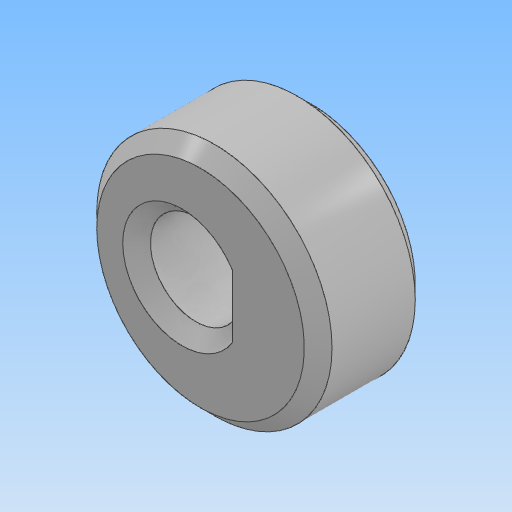
# Autodesk Inventor part: V1_Cycloid_Cam
Saved by Autodesk Inventor 2021 (Build 250183000, 183)
## iProperties
Created: 2020-12-17
Part Number: V1_Cycloid_Cam
Material: PPS Plastic
Document SubType Name: Modeling
Designer: ndevr
Density: 1.637 g/cm^3
Appearance: Smooth - White
Author: ndevr
Autodesk Inventor part; units mm, degrees
ref_plane "Work Plane19" through (-1.0583, 0, 0) normal (1, 0, 0) x (0, 0, 1)
ref_plane "XZ Vertical Span" through (0, 0, 0) normal (0, 1, 0) x (-1, 0, 0)
derived "V1_N17Cycloid_CamShaft.ipt"
sketch "Sketch16" plane through (0, 0, 0) normal (0, 0, 1) x (1, 0, 0)
  circle A0 centre (0, 0) radius 6.7333 construction
  circle A1 centre (0, 0) radius 6.7333
  circle A2 centre (-1.0583, 0) radius 2.5
  line L0 (0.9417, 1.5) -> (0.9417, -1.5)
  circle A3 centre (-1.0583, 0) radius 2.6016
  line L1 (1.0433, 1.5335) -> (1.0433, -1.5335)
ref_plane "Bot Cycoid Bot" through (9.525, 0, 10.5172) normal (0, 0, -1) x (-1, 0, 0)
ref_plane "Bot Cycoid Top" through (9.525, 0, 16.8672) normal (0, 0, -1) x (-1, 0, 0)
ref_plane "Top Cycloid Top" through (9.525, 0, 23.6141) normal (0, 0, -1) x (-1, 0, 0)
ref_plane "Top Cycloid Bot" through (9.525, 0, 17.2641) normal (0, 0, -1) x (-1, 0, 0)
ref_plane "Cam Center Plane" through (9.525, 0, 16.8672) normal (0, 0, -1) x (-1, 0, 0)
extrude "Extrusion13" add sketch "Sketch16" along normal up to surface (6.35 mm away) from surface at 10.5172 contours A1 | L1 A3 A2 | A2 L1 picked at (1.4752, 0.3389)
chamfer "Chamfer7" distance 0.7937 angle 45 6 edges at (-6.7333, 0, 16.8672) (-6.7333, 0, 10.5172) (-3.6599, 0, 16.8672) (-3.6599, 0, 10.5172) (1.0433, 0, 16.8672) (1.0433, 0, 10.5172)
body "Solid7"
